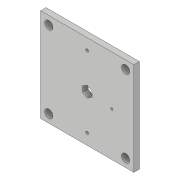
# Autodesk Inventor part: AY
Saved by Autodesk Inventor 2019 (Build 230136000, 136)
## iProperties
Created: 2019-11-16
Part Number: AY
Material: Generic
Document SubType Name: Modeling
Designer: Admin
Density: 1 g/cm^3
Appearance: Default
Author: Admin
Autodesk Inventor part; units mm, degrees
ref_plane "YZ Plane" through (0, 0, 0) normal (1, 0, 0) x (0, 1, 0)
ref_plane "XZ Plane" through (0, 0, 0) normal (0, 1, 0) x (-1, 0, 0)
ref_plane "XY Plane" through (0, 0, 0) normal (0, 0, 1) x (1, 0, 0)
sketch "Sketch1" plane through (0, 0, 0) normal (0, 0, 1) x (1, 0, 0)
  line L0 (0, 0) -> (170, 0)
  line L1 (170, 0) -> (170, 170)
  line L2 (170, 170) -> (0, 170)
  line L3 (0, 170) -> (0, 0)
  dimension "d0" = 170
  dimension "d1" = 170
  constraints: 8 end point, 2 parallel, 1 horizontal, 1 perpendicular
  measures "d0" distance of L2.end L1.end
  measures "d1" distance of L1.end L0.end
extrude "Extrusion1" add sketch "Sketch1" along normal blind 10
sketch "Sketch2" plane through (0, 0, 10) normal (0, 0, 1) x (1, 0, 0)
  line L0 (170, 170) -> (0, 170) projected
  line L1 (0, 170) -> (0, 155)
  line L2 (0, 170) -> (0, 0) projected
  line L3 (0, 0) -> (170, 0) projected
  line L4 (0, 0) -> (0, 15)
  line L5 (0, 15) -> (155, 15)
  line L6 (155, 15) -> (155, 155)
  line L7 (155, 155) -> (15, 155)
  line L8 (15, 155) -> (15, 15)
  line L9 (15, 155) -> (30, 155)
  circle A0 centre (15, 155) radius 7.5
  circle A1 centre (155, 155) radius 7.5
  circle A2 centre (155, 15) radius 7.5
  circle A3 centre (15, 15) radius 7.5
  dimension "d4" = 15
  dimension "d5" = 15
  dimension "d6" = 155
  dimension "d7" = 140
  dimension "d8" = 140
  dimension "d9" = 140
  dimension "d10" = 15
  dimension "d11" = 15
  dimension "d12" = 15
  dimension "d13" = 15
  constraints: 14 end point, 4 centre point, 4 coincident, 4 point on line, 3 perpendicular
  measures "d4" distance of L0.end L1.end
  measures "d5" distance of L2.end L4.end
  measures "d6" distance of L4.end L5.end
  measures "d7" distance of L5.end L6.end
  measures "d8" distance of L6.end L7.end
  measures "d9" distance of L7.end L8.end
  measures "d10" diameter of A0
  measures "d11" diameter of A1
  measures "d12" diameter of A2
  measures "d13" diameter of A3
extrude "Extrusion2" cut sketch "Sketch2" against normal blind 10 contours L8 A3 L5 | L5 A3 | L5 A3 L8 | A2 L6 L5 | L5 L6 A2 | A0 L7 L8 | L8 L7 A0 | A1 L7 L6 | L6 L7 A1
sketch "Sketch3" plane through (0, 0, 10) normal (0, 0, 1) x (1, 0, 0)
  line L0 (170, 170) -> (0, 170) projected
  line L1 (0, 170) -> (85, 170)
  line L2 (85, 170) -> (85, 85)
  line L3 (93.542, 90.1995) -> (93.7739, 80.2022)
  line L4 (93.7739, 80.2022) -> (85.2319, 75.0027)
  line L5 (85.2319, 75.0027) -> (76.458, 79.8005)
  line L6 (76.458, 79.8005) -> (76.2261, 89.7978)
  line L7 (76.2261, 89.7978) -> (84.7681, 94.9973)
  line L8 (84.7681, 94.9973) -> (93.542, 90.1995)
  point P0 (0, 0)
  dimension "d16" = 85
  dimension "d17" = 85
  dimension "d18" = 10
  constraints: 16 end point, 1 coincident, 1 midpoint, 1 perpendicular, 13 other
  measures "d16" distance of L0.end L1.end
  measures "d17" distance of L1.end L2.end
  measures "d18" distance of L7.end L3.start
extrude "Extrusion3" cut sketch "Sketch3" against normal blind 10
sketch "Sketch4" plane through (0, 0, 10) normal (0, 0, 1) x (1, 0, 0)
  line L0 (170, 170) -> (0, 170) projected
  line L1 (0, 170) -> (85, 170)
  line L2 (85, 170) -> (85, 150)
  line L3 (85, 150) -> (85, 20)
  circle A0 centre (85, 150) radius 2.5
  circle A1 centre (85, 20) radius 2.5
  point P0 (0, 0)
  dimension "d21" = 85
  dimension "d22" = 20
  dimension "d23" = 130
  dimension "d24" = 5
  dimension "d25" = 5
  constraints: 6 end point, 2 centre point, 2 coincident, 1 midpoint, 1 perpendicular, 1 point on line
  measures "d21" distance of L0.end L1.end
  measures "d22" distance of L1.end L2.end
  measures "d23" distance of L2.end L3.end
  measures "d24" diameter of A0
  measures "d25" diameter of A1
extrude "Extrusion4" cut sketch "Sketch4" against normal blind 10
sketch "Sketch5" plane through (0, 0, 10) normal (0, 0, 1) x (1, 0, 0)
  line L0 (170, 0) -> (170, 170) projected
  line L1 (170, 0) -> (170, 80)
  line L2 (170, 80) -> (130, 80)
  circle A0 centre (130, 80) radius 2
  point P0 (0, 0)
  dimension "d28" = 80
  dimension "d29" = 40
  dimension "d30" = 4
  constraints: 4 end point, 1 centre point, 1 coincident, 1 perpendicular, 1 point on line
  measures "d28" distance of L0.start L1.end
  measures "d29" distance of L1.end L2.end
  measures "d30" diameter of A0
extrude "Extrusion5" cut sketch "Sketch5" against normal blind 10
body "Solid1"
